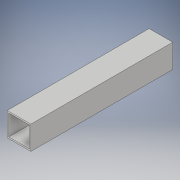
# Autodesk Inventor part: Hook 1st
Saved by Autodesk Inventor 2018 (Build 220112000, 112)
## iProperties
Created: 2020-01-24
Part Number: Hook 1st
Material: Generic
Document SubType Name: Modeling
Designer: s-2513398
Density: 1 g/cm^3
Appearance: Default
Author: s-2513398
Autodesk Inventor part; units mm, degrees
ref_plane "YZ Plane" through (0, 0, 0) normal (1, 0, 0) x (0, 1, 0)
ref_plane "XZ Plane" through (0, 0, 0) normal (0, 1, 0) x (-1, 0, 0)
ref_plane "XY Plane" through (0, 0, 0) normal (0, 0, 1) x (1, 0, 0)
sketch "Sketch1" plane through (0, 0, 0) normal (0, 0, 1) x (1, 0, 0)
  line L0 (0, 0) -> (25.4, 0)
  line L1 (25.4, 0) -> (25.4, 25.4053)
  line L2 (25.4, 25.4053) -> (0, 25.4053)
  line L3 (0, 25.4053) -> (0, 0)
  line L4 (1.5875, 22.2862) -> (1.5875, 23.8178) construction
  line L5 (1.5875, 23.8178) -> (23.8125, 23.8178)
  line L6 (23.8125, 23.8178) -> (23.8125, 1.5875)
  line L7 (23.8125, 1.5875) -> (1.5875, 1.5875)
  line L8 (1.5875, 1.5875) -> (1.5875, 23.8178)
  dimension "d0" = 25.4
  dimension "d4" = 22.225
  constraints: 18 end point, 4 parallel, 2 horizontal, 2 perpendicular, 1 vertical
  measures "d0" distance of L2.end L1.end
  measures "d4" distance of L6.end L7.end
extrude "Extrusion1" add sketch "Sketch1" along normal blind 152.4
body "Solid1"
